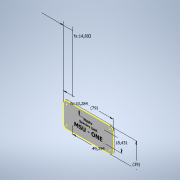
# Autodesk Inventor part: MarkingMSU_ONE
Saved by Autodesk Inventor 2022 (Build 260153000, 153)
## iProperties
Created: 2021-12-10
Part Number: MarkingMSU_ONE
Material: Generic
Document SubType Name: Modeling
Designer: Viktor
Density: 1 g/cm^3
Appearance: Default
Author: Viktor
Autodesk Inventor part; units mm, degrees
ref_plane "YZ Plane" through (0, 0, 0) normal (1, 0, 0) x (0, 1, 0)
ref_plane "XZ Plane" through (0, 0, 0) normal (0, 1, 0) x (-1, 0, 0)
ref_plane "XY Plane" through (0, 0, 0) normal (0, 0, 1) x (1, 0, 0)
sketch "Sketch1" plane through (0, 0, 0) normal (0, 0, 1) x (1, 0, 0)
  line L0 (-39.5, -19.5) -> (39.5, -19.5)
  line L1 (39.5, -19.5) -> (39.5, 19.5)
  line L2 (39.5, 19.5) -> (-39.5, 19.5)
  line L3 (-39.5, 19.5) -> (-39.5, -19.5)
  line L4 (-39.5, -19.5) -> (39.5, 19.5) construction
  line L5 (39.5, -19.5) -> (-39.5, 19.5) construction
  point P0 (0, 0)
  dimension "d0" = 79
  dimension "d1" = 39
  constraints: 12 end point, 2 midpoint, 2 parallel, 1 horizontal, 1 perpendicular
  measures "d0" distance of L1.end L2.end
  measures "d1" distance between parallel lines of L0 L2
extrude "Extrusion1" add sketch "Sketch1" along normal blind 2
fillet "Fillet1" radius 5 4 edges at (39.5, 19.5, 1) (-39.5, 19.5, 1) (39.5, -19.5, 1) (-39.5, -19.5, 1)
sketch "Sketch2" plane through (0, 0, 2) normal (0, 0, 1) x (1, 0, 0)
  line L0 (-24.6971, 9.2157) -> (24.6971, 9.2157) construction
  line L1 (24.6971, 9.2157) -> (24.6971, -9.2157) construction
  line L2 (24.6971, -9.2157) -> (-24.6971, -9.2157) construction
  line L3 (-24.6971, -9.2157) -> (-24.6971, 9.2157) construction
  line L4 (34.5, 19.5) -> (-34.5, 19.5) projected
  line L5 (-34.5, -19.5) -> (34.5, -19.5) projected
  line L6 (-39.5, 14.5) -> (-39.5, -14.5) projected
  line L7 (39.5, -14.5) -> (39.5, 14.5) projected
  arc A0 (-39.5, -14.5) -> (-34.5, -19.5) centre (-34.5, -14.5) ccw projected
  line L8 (-34.5, -19.5) -> (34.5, -19.5) projected
  arc A1 (34.5, -19.5) -> (39.5, -14.5) centre (34.5, -14.5) ccw projected
  line L9 (39.5, -14.5) -> (39.5, 14.5) projected
  arc A2 (39.5, 14.5) -> (34.5, 19.5) centre (34.5, 14.5) ccw projected
  line L10 (34.5, 19.5) -> (-34.5, 19.5) projected
  arc A3 (-34.5, 19.5) -> (-39.5, 14.5) centre (-34.5, 14.5) ccw projected
  line L11 (-39.5, 14.5) -> (-39.5, -14.5) projected
  point P0 (0, 0)
  dimension "d5" = 10.2843
  dimension "d6" = 18.4313
  dimension "d7" = 39
  dimension "d8" = 14.8029
  dimension "d9" = 79
  dimension "d10" = 49.3942
  constraints: 2 other
  measures "d5" distance between parallel lines of L4 L0
  measures "d6" distance between parallel lines of L0 L2
  measures "d7" distance between parallel lines of L5 L4
  measures "d8" distance between parallel lines of L6 L3
  measures "d9" distance between parallel lines of L7 L6
  measures "d10" distance between parallel lines of L1 L3
equation "\"d5\" = -0.5 * d6 + 0.5 * d7"
equation "\"d8\" = -0.5 * d10 + 0.5 * d9"
body "Solid1"
